Autodesk Inventor part; units mm, degrees
(part 2 of 2)
extrude "Extrusion20" cut sketch "Sketch22" against normal blind 10
sketch "Sketch23" plane through (0, 15, 0) normal (0, 1, 0) x (1, 0, 0)
  circle A0 centre (43.0038, 0) radius 3.25 projected
  circle A1 centre (43.0038, 0) radius 5.5
  point P0 (0, 0)
  dimension "d271" = 11
  constraints: 1 centre point, 1 coincident
  measures "d271" diameter of A1
extrude "Extrusion21" cut sketch "Sketch23" against normal blind 6
sketch "Sketch24" plane through (0, 15, 0) normal (0, 1, 0) x (1, 0, 0)
  circle A0 centre (20, 0) radius 9.5 construction
  line L0 (29.5, 0) -> (37.5038, 0) construction
  circle A1 centre (43.0038, 0) radius 5.5 construction
  line L1 (33.5019, 0) -> (33.5019, 5) construction
  line L2 (33.5019, 0) -> (33.5019, -5) construction
  arc A2 (34.5019, 5) -> (32.5019, 5) centre (33.5019, 5) ccw
  arc A3 (32.5019, -5) -> (34.5019, -5) centre (33.5019, -5) ccw
  line L3 (32.5019, 5) -> (32.5019, -5)
  line L4 (34.5019, -5) -> (34.5019, 5)
  point P0 (0, 0)
  dimension "d274" = 5
  dimension "d275" = 5
  dimension "d276" = 2
  constraints: 10 end point, 4 point on circle, 3 tangent, 2 centre point, 2 coincident, 2 horizontal alignment, 2 vertical, 1 horizontal, 1 midpoint, 1 parallel, 2 other
  measures "d274" distance of L1.start L1.end
  measures "d275" distance of L1.start L2.end
  measures "d276" diameter of A2
extrude "Extrusion22" cut sketch "Sketch24" against normal through all
mirror "Mirror5" about plane through (-10, 15, -57.7) normal (-1, 0, 0) of "Extrusion21", "Extrusion22"
sketch "Sketch25" plane through (-63.0038, 15, 0) normal (0, 1, 0) x (1, 0, 0)
  circle A0 centre (0, 0) radius 3.25
  point P0 (63.0038, 0)
  constraints: 1 centre point
extrude "Extrusion23" cut sketch "Sketch25" against normal blind 10
body "Solid1"
